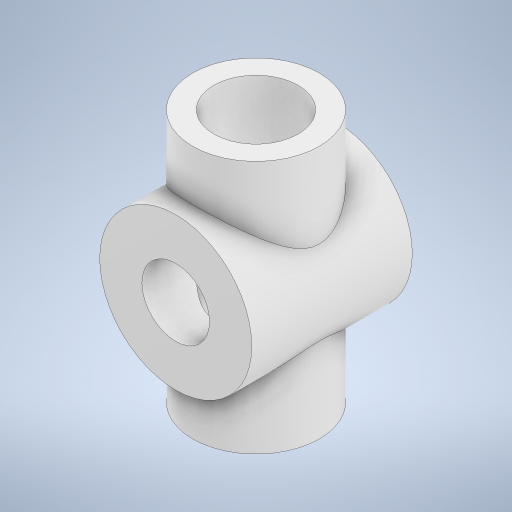
# Autodesk Inventor part: Space
Saved by Autodesk Inventor 2023 (Build 270158030, 158C)
## iProperties
Created: 2022-10-01
Part Number: Space
Material: ABS Plastic
Document SubType Name: Modeling
Designer: cjj5381
Density: 1.06 g/cm^3
Appearance: Smooth - White
Author: cjj5381
Autodesk Inventor part; units mm, degrees
ref_plane "YZ Plane" through (0, 0, 0) normal (1, 0, 0) x (0, 1, 0)
ref_plane "XZ Plane" through (0, 0, 0) normal (0, 1, 0) x (-1, 0, 0)
sketch "Sketch1" plane through (0, 0, 0) normal (0, 1, 0) x (-1, 0, 0)
  line L0 (0, 0) -> (0, -14.3069)
  circle A0 centre (0, 0) radius 5
  circle A1 centre (0, 0) radius 7.5
  dimension "d37" = 10
  dimension "d38" = 15
  constraints: 2 centre point, 2 coincident, 2 end point, 1 vertical
  measures "d37" diameter of A0
  measures "d38" diameter of A1
extrude "Extrusion1" add sketch "Sketch1" along normal mid plane 30
ref_plane "Work Plane2" through (0, 0, 7.5) normal (0, 0, 1) x (1, 0, 0)
sketch "Sketch7" plane through (0, 0, 7.5) normal (0, 0, 1) x (1, 0, 0)
  circle A0 centre (0, 0) radius 7
  point P0 (0, 0)
  dimension "d39" = 14
  constraints: 1 centre point, 1 coincident
  measures "d39" diameter of A0
extrude "Extrusion3" cut sketch "Sketch7" against normal blind 2
sketch "Sketch8" plane through (0, 0, 0) normal (0, 1, 0) x (-1, 0, 0)
  line L0 (0, 0) -> (0, 13.2355)
  circle A0 centre (0, 0) radius 7.5 projected
  line L1 (7, 5.5) -> (7, 9.5)
  line L2 (7, 9.5) -> (9, 9.5)
  line L3 (-5.099, 5.5) -> (5.099, 5.5) projected
  line L4 (5.099, 5.5) -> (7, 5.5)
  line L5 (9, 9.5) -> (9, 0)
  line L6 (9, 0) -> (7.5, 0)
  circle A1 centre (0, 0) radius 7.5 projected
  point P0 (0, 6.6178)
  point P1 (7.1053, 2.4011)
  dimension "d44" = 14
  dimension "d46" = 2
  dimension "d50" = 4
  constraints: 12 end point, 3 point on circle, 3 vertical, 1 horizontal, 1 midpoint, 1 perpendicular, 1 point on line
  measures "d44" diameter of L1 point (0, 6.618)
  measures "d46" distance of L1.end L2.end
  measures "d50" distance of L1.start L1.end
revolve "Revolution1" add sketch "Sketch8" angle 360 about axis through (0, 0, 0) along (0, 0, 1) contours L4 L1 L2 L5 L6 A0
mirror "Mirror3" about plane through (0, 0, 0) normal (0, 0, 1) of "Revolution1", "Extrusion3"
sketch "Sketch9" plane through (0, -15, 0) normal (0, -1, 0) x (1, 0, 0)
  circle A0 centre (0, 0) radius 5
  circle A1 centre (0, 0) radius 5 projected
  constraints: 1 centre point, 1 coincident, 1 concentric
extrude "Extrusion4" cut sketch "Sketch9" against normal through all
sketch "Sketch10" plane through (0, 0, 5.5) normal (0, 0, 1) x (1, 0, 0)
  circle A0 centre (0, 0) radius 7 projected
  constraints: 1 coincident
hole "Hole4" at (0, 0, 5.5) direction (0, 0, -1) diameter 8.001 end through all
sketch "Sketch11" plane through (0, 0, 5.5) normal (0, 0, 1) x (1, 0, 0)
  circle A0 centre (0, 0) radius 7
  circle A1 centre (0, 0) radius 4.0005
  constraints: 2 centre point, 2 coincident
extrude "Extrusion5" add sketch "Sketch11" along normal up to surface (4 mm away)
body "Solid1"
